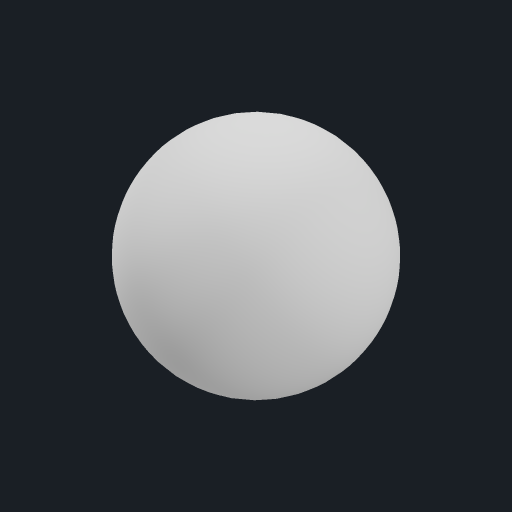
# Autodesk Inventor part: kula
Saved by Autodesk Inventor 2023.4 (Build 274418000, 418)
## iProperties
Created: 2024-04-25
Part Number: kula
Material: Generic
Document SubType Name: Modeling
Designer: figa3
Mass: 1000 g
Surface Area: 28.2743 cm^2
Volume: 14.1372 cm^3
Density: 70.7355 g/cm^3
Appearance: Default
Author: figa3
Autodesk Inventor part; units mm, degrees
ref_plane "YZ Plane" through (0, 0, 0) normal (1, 0, 0) x (0, 1, 0)
ref_plane "XZ Plane" through (0, 0, 0) normal (0, 1, 0) x (-1, 0, 0)
ref_plane "XY Plane" through (0, 0, 0) normal (0, 0, 1) x (1, 0, 0)
sketch "Sketch1" plane through (0, 0, 0) normal (0, 1, 0) x (-1, 0, 0)
  circle A0 centre (0, 0) radius 15
  line L0 (15, 0) -> (-15, 0)
  dimension "d0" = 30
  constraints: 2 end point, 2 point on circle, 1 centre point, 1 coincident, 1 horizontal
  measures "d0" diameter of A0
revolve "Revolution1" add sketch "Sketch1" angle 360 about axis through (-15, 0, 0) along (1, 0, 0) picked at (-4.4273, -2.3236) contours A0 L0
body "Solid1"
